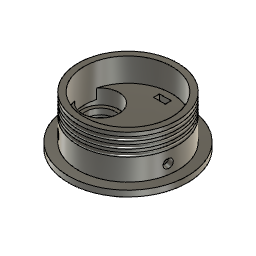
Connector bottom cap v34 (Autodesk Fusion 360 design; units mm, degrees)
Autodesk Fusion 360 part; units mm, degrees
note: some values were not read from the file. Set by a fixed rule: which sketch regions a step uses.
sketch "Sketch1" plane through (0, 0, 0) normal (0, 0, 1) x (1, 0, 0)
  circle A0 centre (0, 0) radius 36
  dimension "d1" = 72
  constraint coincident A0.centre origin
  measures "d1" diameter of A0
extrude "Extrude1" add sketch "Sketch1" along normal blind 10
sketch "Sketch2" plane through (0, 0, 10) normal (0, 0, 1) x (-1, 0, 0)
  circle A0 centre (0, 0) radius 36
  circle A1 centre (0, 0) radius 33.5
  dimension "d5" = -2.5
extrude "Extrude2" cut sketch "Sketch2" against normal blind 7 contours A1
sketch "Sketch4" plane through (0, 0, 3) normal (0, 0, 1) x (-1, 0, 0)
  circle A0 centre (0, 0) radius 25.25
  circle A1 centre (0, 0) radius 22.25
  circle A2 centre (0, 0) radius 33.5
  dimension "d11" = 50.5
  dimension "d12" = 44.5
  constraint coincident A0.centre A1.centre
  measures "d11" diameter of A0
  measures "d12" diameter of A1
extrude "Extrude4" add sketch "Sketch4" along normal blind 2.5 contours A0
sketch "Sketch5" plane through (0, 0, 3) normal (0, 0, 1) x (-1, 0, 0)
  circle A0 centre (0, 0) radius 22.25
  circle A1 centre (0, 0) radius 21
  line L0 (0, 0) -> (-14, 0)
  line L1 (-17.4668, -11.658) -> (-17.4668, -10)
  line L2 (-16.4924, -13) -> (16.4924, -13)
  line L3 (-16.4924, 13) -> (16.4924, 13)
  line L4 (0, -13) -> (0, -21)
  line L5 (0, -13) -> (-15, -13)
  spline S0 degree 5 poles (-15, -13) (-14.8666, -13.2826) (-14.5692, -13.8414) (-14.0314, -14.6603) (-13.143, -15.7044) (-11.8108, -16.8822) (-10.331, -17.8796) (-8.7699, -18.6586) (-7.1673, -19.2229) (-5.5223, -19.639) (-3.8099, -20.0024) (-2.3567, -20.3324) (-1.2046, -20.6389) (-0.4065, -20.8744) (0, -21) knots 0 0 0 0 0 0 0.1 0.2 0.3 0.4 0.5 0.6 0.7 0.8 0.9 1 1 1 1 1 1
  spline S1 degree 5 poles (15, -13) (14.8666, -13.2826) (14.5692, -13.8414) (14.0314, -14.6603) (13.143, -15.7044) (11.8108, -16.8822) (10.331, -17.8796) (8.7699, -18.6586) (7.1673, -19.2229) (5.5223, -19.639) (3.8099, -20.0024) (2.3567, -20.3324) (1.2046, -20.6389) (0.4065, -20.8744) (0, -21) knots 0 0 0 0 0 0 0.1 0.2 0.3 0.4 0.5 0.6 0.7 0.8 0.9 1 1 1 1 1 1
  line L6 (-15.6363, -11.6523) -> (-14.3637, -14.3477)
  line L7 (-1.862, -20.4249) -> (1.862, -21.5751)
  line L8 (15.6363, -11.6523) -> (14.3637, -14.3477)
  line L9 (1.862, -20.4249) -> (-1.862, -21.5751)
  spline S2 degree 5 poles (15, 13) (14.8666, 13.2826) (14.5692, 13.8414) (14.0314, 14.6603) (13.143, 15.7044) (11.8108, 16.8822) (10.331, 17.8796) (8.7699, 18.6586) (7.1673, 19.2229) (5.5223, 19.639) (3.8099, 20.0024) (2.3567, 20.3324) (1.2046, 20.6389) (0.4065, 20.8744) (0, 21) knots 0 0 0 0 0 0 0.1 0.2 0.3 0.4 0.5 0.6 0.7 0.8 0.9 1 1 1 1 1 1
  line L10 (15.6363, 11.6523) -> (14.3637, 14.3477)
  line L11 (1.862, 20.4249) -> (-1.862, 21.5751)
  spline S3 degree 5 poles (-15, 13) (-14.8666, 13.2826) (-14.5692, 13.8414) (-14.0314, 14.6603) (-13.143, 15.7044) (-11.8108, 16.8822) (-10.331, 17.8796) (-8.7699, 18.6586) (-7.1673, 19.2229) (-5.5223, 19.639) (-3.8099, 20.0024) (-2.3567, 20.3324) (-1.2046, 20.6389) (-0.4065, 20.8744) (0, 21) knots 0 0 0 0 0 0 0.1 0.2 0.3 0.4 0.5 0.6 0.7 0.8 0.9 1 1 1 1 1 1
  line L12 (-15.6363, 11.6523) -> (-14.3637, 14.3477)
  line L13 (-1.862, 20.4249) -> (1.862, 21.5751)
  point P0 (-9, -18.5)
  point P1 (9, -18.5)
  point P2 (9, 18.5)
  point P3 (-9, 18.5)
  dimension "d15" = 42
  dimension "d18" = 14
  dimension "d23" = 8
  dimension "d24" = 15
  constraint coincident A0.centre A1.centre
  constraint horizontal L0
  constraint perpendicular L0 L1
  constraint coincident A1 L1.start
  constraint coincident A1 L2.start
  constraint coincident A1 L2.end
  constraint symmetric L0 L2.start L3.start
  constraint symmetric L0 L2.end L3.end
  constraint midpoint L2 L4.start
  constraint coincident A1 L4.end
  constraint perpendicular L2 L4
  constraint perpendicular L4 L5
  constraint midpoint L5.end L6
  constraint midpoint L4.end L7
  constraint symmetric S0.end L4 S1.end
  constraint symmetric L4 L5.end S1.start
  constraint symmetric L4 P0 P1
  constraint symmetric L4 L6.start L8.start
  constraint symmetric L4 L6.end L8.end
  constraint symmetric L4 L7.start L9.start
  constraint symmetric L4 L7.end L9.end
  constraint symmetric L0 L4.end S2.end
  constraint symmetric L0 L5.end S3.start
  constraint symmetric L0 P0 P3
  constraint symmetric L0 S1.start S2.start
  constraint symmetric L0 P1 P2
  constraint symmetric L0 L6.start L12.start
  constraint symmetric L0 L6.end L12.end
  constraint symmetric L0 L7.start L13.start
  constraint symmetric L0 L7.end L13.end
  constraint symmetric L0 L8.start L10.start
  constraint symmetric L0 L8.end L10.end
  constraint symmetric L0 L9.start L11.start
  constraint symmetric L0 L9.end L11.end
  measures "d15" diameter of A1
  measures "d18" distance of A0.centre L0.end
  measures "d23" distance of L4.start L4.end
  measures "d24" distance of L4.start L5.end
extrude "Extrude5" add sketch "Sketch5" against normal blind 10 contours L3 S2 S3 | L2 L4 L5 S0 | L2 L4 S1
extrude "Extrude6" add 1 faces at (-24.0732, 2.3598, 5.5) along direction (0, 0, 1) blind 5
sketch "Sketch6" plane through (0, 0, 3) normal (0, 0, 1) x (-1, 0, 0)
  circle A0 centre (0, 0) radius 25.75
  circle A1 centre (0, 0) radius 30.25
  circle A2 centre (0, 0) radius 33.5
  circle A3 centre (0, 0) radius 25.25
  dimension "d25" = 51.5
  dimension "d26" = 4.5
  measures "d25" diameter of A0
extrude "Extrude7" add 1 faces at (-30.6253, 1.6643, 3) along direction (0, 0, 1) blind 7
extrude "Extrude8" cut sketch "Sketch6" along normal blind 7 contours A1
extrude "Extrude9" cut 1 faces at (-23.9781, -8.735, 10) along direction (0, 0, -1) blind 7
sketch "Sketch7" plane through (0, 0, 3) normal (0, 0, 1) x (-1, 0, 0)
  circle A0 centre (0, 0) radius 22.25
  circle A1 centre (14, 0) radius 7.5
  line L0 (0, 0) -> (-13, 0)
  line L1 (-13, 0) -> (-13, -16)
  circle A2 centre (-9.7282, -9.2513) radius 7.5
  circle A3 centre (-9.7282, 9.2513) radius 7.5
  dimension "d33" = 14
  dimension "d34" = 13
  dimension "d36" = 15
  dimension "d49" = 16
  dimension "d51" = 15
  constraint coincident A0.centre L0.start
  constraint horizontal L0
  constraint perpendicular L0 L1
  constraint coincident L1.end A2
  constraint symmetric L0 A2 A3
  measures "d33" distance of A0.centre A1.centre
  measures "d34" distance of A0.centre L0.end
  measures "d36" diameter of A1
  measures "d49" distance of L0.end L1.end
  measures "d51" diameter of A2
extrude "Extrude10" cut sketch "Sketch7" against normal blind 15 contours A1
extrude "Extrude11" cut 1 faces at (-24.0732, 2.3598, 10.5) along direction (0, 0, -1) blind 0.5
sketch "Sketch9" plane through (0, -13, 0) normal (0, 1, 0) x (-1, 0, 0)
  line L0 (15, 0) -> (-15, 0)
  line L1 (-15, -7) -> (15, -7)
  line L2 (15, -7) -> (15, 0)
  circle A0 centre (0, -4) radius 1.75
  line L3 (-15, 0) -> (-15, -7)
  dimension "d44" = 3.5
  measures "d44" diameter of A0
extrude "Extrude13" cut sketch "Sketch9" against normal blind 4 contours A0
sketch "Sketch10" plane through (0, 0, 3) normal (0, 0, 1) x (-1, 0, 0)
  circle A0 centre (14, 0) radius 7.5
  circle A1 centre (0, 0) radius 22.25
  circle A2 centre (0, 17) radius 3
  dimension "d47" = 6
  dimension "d48" = 17
  measures "d47" diameter of A2
  measures "d48" distance of A1.centre A2.centre
extrude "Extrude14" cut sketch "Sketch10" against normal blind 9 contours A2
sketch "Sketch11" plane through (0, 13, 0) normal (0, -1, 0) x (1, 0, 0)
  line L0 (15, 0) -> (-15, 0)
  line L1 (-15, 0) -> (-15, -7)
  line L2 (-15, -7) -> (15, -7)
  circle A0 centre (0, -4) radius 2.5
  line L3 (15, -7) -> (15, 0)
  dimension "d56" = 5
  measures "d56" diameter of A0
extrude "Extrude15" cut sketch "Sketch11" against normal blind 4 contours A0
sketch "Sketch12" plane through (0, 0, 3) normal (0, 0, 1) x (-1, 0, 0)
  circle A0 centre (0, 17) radius 3
  circle A1 centre (14, 0) radius 7.5
  circle A2 centre (0, 0) radius 22.25
  line L0 (0, 0) -> (0, -17)
  line L1 (3, -19) -> (-3, -19)
  line L2 (-3, -19) -> (-3, -16)
  line L3 (-3, -16) -> (3, -16)
  line L4 (3, -16) -> (3, -19)
  dimension "d59" = 17
  constraint coincident A2.centre L0.start
  constraint vertical L0
  constraint horizontal L1
  constraint vertical L2
  constraint horizontal L3
  constraint vertical L4
  measures "d59" distance of A2.centre L0.end
extrude "Extrude16" cut sketch "Sketch12" against normal blind 9 contours L1 L2 L3 L4
extrude "Extrude17" add 1 faces at (-24.0732, 2.3598, 10) along direction (0, 0, 1) blind 10
sketch "Sketch13" plane through (0, 0, 0) normal (1, 0, 0) x (0, 1, 0)
  line L0 (25.5, 20.0277) -> (25.5, 10)
  line L1 (0, 20) -> (25.25, 20)
  line L2 (25.25, 20) -> (25.25, 10)
  circle A0 centre (25.25, 15) radius 1
  dimension "d87" = 25.25
  dimension "d88" = 2
  constraint vertical L0
  constraint perpendicular L0 L1
  constraint perpendicular L1 L2
  constraint midpoint L2 A0.centre
  measures "d87" distance of L1.start L1.end
  measures "d88" diameter of A0
revolve "Revolve1" cut sketch "Sketch13" angle 360 about axis through (0, 0, 10) along (0, 0, 1) contours L2 A0
extrude "Extrude18" cut 1 faces at (-23.1078, -24.9626, 10) along direction (0, 0, -1) blind 10
extrude "Extrude19" add 1 faces at (5.9496, 7.4228, 3) along direction (0, 0, 1) blind 5
ref_plane "WorkPlane1" through (-16.2304, -19.3426, 5.9475) normal (-0.642788, -0.766044, 0) x (-0.766044, 0.642788, 0)
sketch "Sketch14" plane through (-16.2304, -19.3426, 5.9767) normal (-0.642788, -0.766044, 0) x (-0.766044, 0.642788, 0)
  circle A0 centre (0, -2) radius 2.25
  dimension "d84" = 4.5
  measures "d84" diameter of A0
extrude "Extrude20" cut sketch "Sketch14" against normal blind 3
pattern_circular "C-Pattern1" count 3 over 360 about axis through (0, 0, 3) along (0, 0, 1) of "Extrude20"
sketch "Sketch15" plane through (0, 0, 0) normal (0, 0, -1) x (1, 0, 0)
  circle A0 centre (0, 0) radius 30.25
  circle A1 centre (-14, 0) radius 7.5
  spline S0 degree 3 poles (15, -13) (14.4931, -14.0736) (13.7828, -14.9655) (12.1032, -16.6739) (10.8137, -17.6578) (7.7378, -19.0884) (6.3476, -19.4388) (3.4035, -20.1032) (1.9748, -20.39) (0, -21) knots 0 0 0 0 0.35618 0.35618 0.856977 0.856977 1.292786 1.292786 1.730402 1.730402 1.730402 1.730402
  spline S1 degree 3 poles (0, -21) (-3.8794, -19.8017) (-6.1448, -19.7015) (-10.3003, -17.9598) (-11.5145, -17.1003) (-12.9609, -15.8282) (-13.4716, -15.2991) (-14.3389, -14.195) (-14.7083, -13.6179) (-15, -13) knots 0 0 0 0 1.218084 1.218084 2.002702 2.002702 2.474783 2.474783 2.918729 2.918729 2.918729 2.918729
  line L0 (-15, -13) -> (15, -13)
  spline S2 degree 3 poles (0, 21) (3.8794, 19.8017) (6.1448, 19.7015) (10.3003, 17.9598) (11.5145, 17.1003) (12.9609, 15.8282) (13.4716, 15.2991) (14.3389, 14.195) (14.7083, 13.6179) (15, 13) knots 0 0 0 0 1.218084 1.218084 2.002702 2.002702 2.474783 2.474783 2.918729 2.918729 2.918729 2.918729
  line L1 (15, 13) -> (-15, 13)
  spline S3 degree 3 poles (-15, 13) (-14.4931, 14.0736) (-13.7828, 14.9655) (-12.1032, 16.6739) (-10.8137, 17.6578) (-7.7378, 19.0884) (-6.3476, 19.4388) (-3.4035, 20.1032) (-1.9748, 20.39) (0, 21) knots 0 0 0 0 0.35618 0.35618 0.856977 0.856977 1.292786 1.292786 1.730402 1.730402 1.730402 1.730402
  circle A2 centre (-14, 0) radius 9.375
  circle A3 centre (9.9185, -9.7147) radius 9.25
  circle A4 centre (9.9185, 9.7147) radius 9.25
  dimension "d77" = 18.75
  dimension "d85" = 18.5
  dimension "d86" = 18.5
  constraint concentric A1 A2
  measures "d77" diameter of A2
  measures "d85" diameter of A3
  measures "d86" diameter of A4
extrude "Extrude21" cut sketch "Sketch15" against normal blind 2.5 contours A2
sketch "Sketch16" plane through (0, 0, 8) normal (0, 0, 1) x (-1, 0, 0)
  line L0 (-3, -19) -> (-3, -16)
  line L1 (-3, -16) -> (3, -16)
  line L2 (3, -16) -> (3, -19)
  line L3 (3, -19) -> (-3, -19)
  circle A0 centre (0, 17) radius 3
  circle A1 centre (14, 0) radius 7.5
  circle A2 centre (14, 0) radius 9.375
  arc A3 (7.6099, -20.9082) -> (14.302, 17.0445) centre (0, 0) ccw
  arc A4 (-21.912, 3.8637) -> (7.6099, -20.9082) centre (0, 0) ccw
  arc A5 (14.302, 17.0445) -> (-21.912, 3.8637) centre (0, 0) ccw
  dimension "d80" = 18.75
  constraint concentric A1 A2
  measures "d80" diameter of A2
extrude "Extrude22" cut sketch "Sketch16" against normal blind 2.5 contours A2 A3 | A2 A3
extrude "Extrude23" add 1 faces at (6.1848, 8.8426, 8) along direction (0, 0, 1) blind 5
extrude "Extrude24" add 1 faces at (-24.0732, 2.3598, 20) along direction (0, 0, 1) blind 5
pattern_linear "R-Pattern1" count 3 spacing 3.5 along (0, 0, 1) of "Revolve1"
equation "d87 = ( 50.5 / 2 ) * 1 mm"
